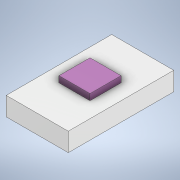
# Autodesk Inventor part: led
Saved by Autodesk Inventor 2022 (Build 260153000, 153)
## iProperties
Created: 2025-05-05
Part Number: led
Material: Ogólny
Document SubType Name: Modeling
Designer: Olga Kowalczyk IB 240875
Density: 1 g/cm^3
Appearance: Domyślna
Author: Olga Kowalczyk IB 240875
Autodesk Inventor part; units mm, degrees
ref_plane "YZ Plane" through (0, 0, 0) normal (1, 0, 0) x (0, 1, 0)
ref_plane "XZ Plane" through (0, 0, 0) normal (0, 1, 0) x (-1, 0, 0)
ref_plane "XY Plane" through (0, 0, 0) normal (0, 0, 1) x (1, 0, 0)
sketch "Szkic1" plane through (0, 0, 0) normal (0, 1, 0) x (-1, 0, 0)
  line L0 (0, 0) -> (10, 0)
  line L1 (10, 0) -> (10, -17)
  line L2 (10, -17) -> (0, -17)
  line L3 (0, -17) -> (0, 0)
  line L4 (7.5, -6) -> (2.5, -6)
  line L5 (2.5, -6) -> (2.5, -11)
  line L6 (2.5, -11) -> (7.5, -11)
  line L7 (7.5, -11) -> (7.5, -6)
  dimension "d0" = 10
  dimension "d1" = 17
  dimension "d2" = 5
  dimension "d3" = 5
  dimension "d4" = 2.5
  dimension "d5" = 6
  constraints: 16 end point, 4 parallel, 2 horizontal, 2 perpendicular
  measures "d0" distance of L1.end L2.end
  measures "d1" distance of L0.end L1.end
  measures "d2" distance of L6.end L5.end
  measures "d3" distance of L5.end L4.end
  measures "d4" distance between parallel lines of L1 L7
  measures "d5" distance between parallel lines of L2 L6
extrude "Wyciągnięcie proste1" add sketch "Szkic1" along normal blind 3
extrude "Wyciągnięcie proste2" add sketch "Szkic1" along normal blind 4 contours L7 L6 L5 L4
